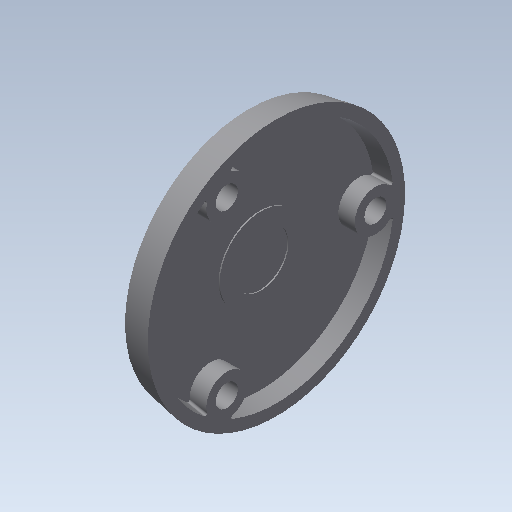
# Autodesk Inventor part: Prop Mount
Saved by Autodesk Inventor 2020 (Build 240152000, 152)
## iProperties
Created: 2013-05-04
Part Number: Prop Mount
Material: Generic
Document SubType Name: Modeling
Designer: John
Density: 1 g/cm^3
Appearance: Default
Author: John
Autodesk Inventor part; units mm, degrees
ref_plane "YZ Plane" through (0, 0, 0) normal (1, 0, 0) x (0, 1, 0)
ref_plane "XZ Plane" through (0, 0, 0) normal (0, 1, 0) x (-1, 0, 0)
ref_plane "XY Plane" through (0, 0, 0) normal (0, 0, 1) x (1, 0, 0)
sketch "Sketch1" plane through (0, 0, 0) normal (1, 0, 0) x (0, 1, 0)
  circle A0 centre (0, 0) radius 28.575
  dimension "d2" = 57.15
  constraints: 1 centre point, 1 coincident
  measures "d2" diameter of A0
extrude "Extrusion1" add sketch "Sketch1" along normal blind 6.35 draft 10
shell "Shell1" thickness 2.54 removed faces 1 at (6.35, -7.4089, 1.8261)
sketch "Sketch2" plane through (2.54, 0, 0) normal (1, 0, 0) x (0, 0, -1)
  circle A0 centre (0, 0) radius 26.4437 projected
  circle A1 centre (22.86, 0) radius 4.7625
  dimension "d4" = 22.86
  dimension "d5" = 9.525
  constraints: 1 centre point
  measures "d4" distance of A0.centre A1.centre
  measures "d5" diameter of A1
extrude "Extrusion2" add sketch "Sketch2" along normal up to surface (3.81 mm away) contours A0 A1 | A0 A1 picked at (20.904, 0) picked at (26.7982, 0.6846)
fillet "Fillet1" radius 0.3969 2 edges at (4.4522, 2.9217, -26.621) (4.4522, -2.9217, -26.621)
pattern_circular "Circular Pattern1" count 3 over 360 about axis through (0.4411, 0, 0) along (1, 0, 0) of "Fillet1", "Extrusion2"
sketch "Sketch5" plane through (2.54, 0, -22.86) normal (1, 0, 0) x (0, 0, -1)
  arc A0 (-38.4225, 17.543) -> (-38.4225, -17.543) centre (-22.86, 0) ccw
  circle A1 centre (-22.86, 0) radius 9.525
  circle A2 centre (-22.86, 0) radius 6.35
  arc A3 (-39.6895, 20.397) -> (-39.6895, -20.397) centre (-22.86, 0) ccw projected
  point P0 (-37.4774, 21.6017)
  point P1 (-37.4774, -21.6017)
  dimension "d18" = 19.05
  dimension "d19" = 3.175
  constraints: 3 centre point, 3 coincident, 2 point on circle, 1 other
  measures "d18" diameter of A1
  measures "d19" radial gap between concentric circles of A1 A2
extrude "Extrusion4" add sketch "Sketch5" along normal blind 0.254
sketch "Sketch6" plane through (6.35, 0, 0) normal (1, 0, 0) x (0, 0, -1)
  arc A0 (-16.0476, 20.9631) -> (-10.1307, 24.3792) centre (-11.43, 19.7973) ccw projected
  arc A1 (26.1784, 3.4161) -> (26.1784, -3.4161) centre (22.86, 0) ccw projected
  arc A2 (-10.1307, -24.3792) -> (-16.0476, -20.9631) centre (-11.43, -19.7973) ccw projected
hole "Hole1" at (6.35, 19.7973, 11.43) at (6.35, 0, -22.86) at (6.35, -19.7973, 11.43) direction (-1, 0, 0) diameter 5.1054 end through all clearance for "Flat Head Machine Screw (82)" size "#10" standard "Ansi Unified Screw Threads"
sketch "Sketch7" plane through (0, 0, 0) normal (-1, 0, 0) x (0, 0, 1)
  circle A0 centre (0, 0) radius 28.575 projected
  line L0 (-0.127, 2.54) -> (0.127, 2.54)
  line L1 (0.127, 2.54) -> (0.127, 12.7)
  line L2 (0.127, 12.7) -> (-0.127, 12.7)
  line L3 (-0.127, 12.7) -> (-0.127, 2.54)
  dimension "d29" = 10.16
  dimension "d30" = 0.254
  dimension "d31" = 2.54
  dimension "d32" = 0.127
  constraints: 8 end point, 2 parallel, 1 horizontal, 1 perpendicular
  measures "d29" distance of L2.end L0.start
  measures "d30" distance of L0.start L0.end
  measures "d31" distance from line of A0.centre L0
  measures "d32" distance from line of A0.centre L3
extrude "Extrusion5" add sketch "Sketch7" along normal blind 0.0254 contours L3 L2 L1 L0
pattern_circular "Circular Pattern2" count 42 over 360 about axis through (0, 0, 0) along (1, 0, 0) of "Extrusion5"
sketch "Sketch8" plane through (0, 0, 0) normal (-1, 0, 0) x (0, 0, 1)
  circle A0 centre (-22.86, 0) radius 2.5527 projected
  circle A1 centre (-17.78, 0) radius 1.5875
  dimension "d38" = 3.175
  dimension "d39" = 5.08
  constraints: 1 centre point
  measures "d38" diameter of A1
  measures "d39" distance of A1.centre A0.centre
extrude "Extrusion6" add sketch "Sketch8" along normal blind 3.175 contours A1
pattern_circular "Circular Pattern3" count 3 over 360 about axis through (0, 0, 0) along (1, 0, 0) of "Extrusion6"
equation "\"d32\" = 0.5 * d30"
body "Solid1"
